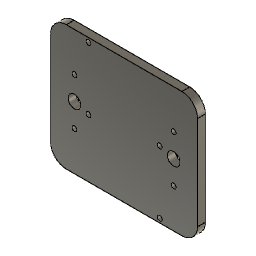
testBaseRig v1 (Autodesk Fusion 360 design; units mm, degrees)
Autodesk Fusion 360 part; units mm, degrees
sketch "Sketch1" plane through (0, 0, 0) normal (0, 1, 0) x (1, 0, 0)
  line L0 (-20.75, -20) -> (20.75, -20) construction
  line L1 (20.75, -20) -> (20.75, 20) construction
  line L2 (20.75, 20) -> (-20.75, 20) construction
  line L3 (-20.75, 20) -> (-20.75, -20) construction
  line L4 (-20.75, -20) -> (20.75, 20) construction
  line L5 (20.75, -20) -> (-20.75, 20) construction
  circle A0 centre (-31.75, 0) radius 4.05
  circle A1 centre (31.75, 0) radius 4.05
  line L6 (25.5, 0) -> (-25.5, 0)
  line L7 (22.803, -2.697) -> (-22.803, -2.697)
  line L8 (-22.803, -2.697) -> (-22.803, -37.303)
  line L9 (-22.803, -37.303) -> (22.803, -37.303)
  line L10 (22.803, -37.303) -> (22.803, -2.697)
  line L11 (22.803, -2.697) -> (-22.803, -37.303) construction
  line L12 (-22.803, -2.697) -> (22.803, -37.303) construction
  line L13 (22.803, 2.697) -> (-22.803, 2.697)
  line L14 (-22.803, 2.697) -> (-22.803, 37.303)
  line L15 (-22.803, 37.303) -> (22.803, 37.303)
  line L16 (22.803, 37.303) -> (22.803, 2.697)
  line L17 (22.803, 2.697) -> (-22.803, 37.303) construction
  line L18 (-22.803, 2.697) -> (22.803, 37.303) construction
  circle A2 centre (-22.803, -37.303) radius 1.55
  circle A3 centre (22.803, -2.697) radius 1.55
  circle A4 centre (-22.803, 2.697) radius 1.55
  circle A5 centre (22.803, 37.303) radius 1.55
  circle A6 centre (-31.75, -15) radius 1.55
  circle A7 centre (-31.75, 15) radius 1.55
  circle A8 centre (31.75, -15) radius 1.55
  circle A9 centre (31.75, 15) radius 1.55
  line L19 (-47, -40) -> (47, -40)
  line L20 (47, -40) -> (47, 40)
  line L21 (47, 40) -> (-47, 40)
  line L22 (-47, 40) -> (-47, -40)
  line L23 (-47, -40) -> (47, 40) construction
  line L24 (47, -40) -> (-47, 40) construction
  point P0 (0, -20)
  point P1 (0, 20)
  point P2 (0, -20)
  point P3 (0, 20)
  dimension "d1" = 41.5
  dimension "d2" = 40
  dimension "d3" = 8.1
  dimension "d4" = 8.1
  dimension "d5" = 11
  dimension "d6" = 11
  dimension "d7" = 51
  dimension "d8" = 20
  dimension "d9" = 20
  dimension "d10" = 45.606
  dimension "d11" = 34.606
  dimension "d12" = 45.606
  dimension "d13" = 34.606
  dimension "d14" = 3.1
  dimension "d15" = 3.1
  dimension "d16" = 3.1
  dimension "d17" = 3.1
  dimension "d18" = 3.1
  dimension "d19" = 3.1
  dimension "d20" = 3.1
  dimension "d21" = 3.1
  dimension "d22" = 15
  dimension "d23" = 15
  dimension "d24" = 15
  dimension "d25" = 15
  dimension "d26" = 94
  dimension "d27" = 80
  constraint horizontal L0
  constraint perpendicular L0 L1
  constraint parallel L0 L2
  constraint parallel L1 L3
  constraint coincident L4 origin
  constraint coincident L5 origin
  constraint perpendicular L3 L6
  constraint midpoint origin L6
  constraint horizontal L7
  constraint perpendicular L7 L8
  constraint parallel L7 L9
  constraint parallel L8 L10
  constraint coincident L11 P2
  constraint coincident L12 P2
  constraint coincident P2 P0
  constraint horizontal L13
  constraint perpendicular L13 L14
  constraint parallel L13 L15
  constraint parallel L14 L16
  constraint coincident L17 P3
  constraint coincident L18 P3
  constraint coincident P3 P1
  constraint coincident L8.end L9.start
  constraint coincident L7.start L10.end
  constraint coincident L13.end L14.start
  constraint coincident L15.end L16.start
  constraint horizontal L19
  constraint perpendicular L19 L20
  constraint parallel L19 L21
  constraint parallel L20 L22
  constraint coincident L23 origin
  constraint coincident L24 origin
  measures "d1" distance of L1.end L2.end
  measures "d2" distance of L0.end L1.end
  measures "d3" diameter of A0
  measures "d4" diameter of A1
  measures "d5" distance of L1 A1.centre
  measures "d6" distance of L3 A0.centre
  measures "d7" distance of L6.start L6.end
  measures "d8" distance of origin P2
  measures "d9" distance of origin P3
  measures "d10" distance of L8.end L9.end
  measures "d11" distance of L7.end L8.end
  measures "d12" distance of L14.end L15.end
  measures "d13" distance of L13.end L14.end
  measures "d14" diameter of A2
  measures "d15" diameter of A3
  measures "d16" diameter of A4
  measures "d17" diameter of A5
  measures "d18" diameter of A6
  measures "d19" diameter of A7
  measures "d20" diameter of A8
  measures "d21" diameter of A9
  measures "d22" distance of A1.centre A8.centre
  measures "d23" distance of A1.centre A9.centre
  measures "d24" distance of A0.centre A7.centre
  measures "d25" distance of A0.centre A6.centre
  measures "d26" distance of L20.end L21.end
  measures "d27" distance of L19.end L20.end
extrude "Extrude1" add sketch "Sketch1" along normal blind 5 contours L7 L8 L9 L10 A2 A3 | L13 L14 L15 L16 A4 A5 | L19 L20 L21 L22
fillet "Fillet1" radius 10 4 edges at (47, 2.5, 40) (47, 2.5, -40) (-47, 2.5, 40) (-47, 2.5, -40)
equation "d6 = d5"
equation "d23 = d22"
equation "d24 = d23"
equation "d25 = d22"
